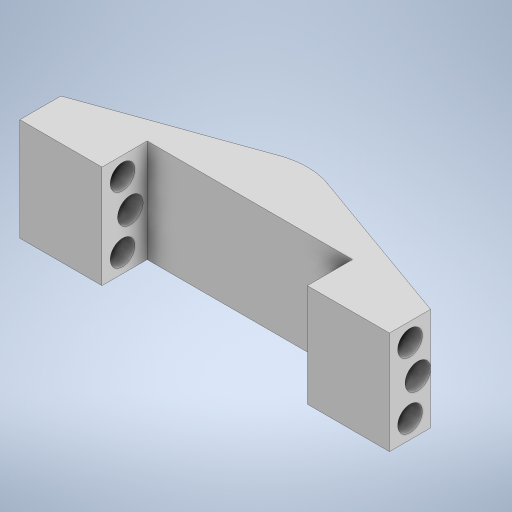
# Autodesk Inventor part: Schieber
Saved by Autodesk Inventor 2024 (Build 280153000, 153)
## iProperties
Created: 2023-08-23
Part Number: Schieber
Material: Generisch
Document SubType Name: Modeling
Designer: rapp
Density: 1 g/cm^3
Appearance: Vorgabe
Author: rapp
Autodesk Inventor part; units mm, degrees
ref_plane "YZ Plane" through (0, 0, 0) normal (1, 0, 0) x (0, 1, 0)
ref_plane "XZ Plane" through (0, 0, 0) normal (0, 1, 0) x (-1, 0, 0)
ref_plane "XY Plane" through (0, 0, 0) normal (0, 0, 1) x (1, 0, 0)
sketch "Skizze1" plane through (0, 0, 0) normal (0, 0, 1) x (1, 0, 0)
  line L0 (-63, 0) -> (63, 0) projected
  line L1 (0, -6) -> (0, 18.5) projected
  arc A0 (5.8901, 13.979) -> (-5.8901, 13.979) centre (0, -2.5) ccw
  line L2 (-5.8901, 13.979) -> (-45, 0)
  line L3 (5.8901, 13.979) -> (45, 0)
  line L4 (-45, 0) -> (45, 0)
  dimension "d2" = 35
  dimension "d3" = 15
  dimension "d4" = 45
  constraints: 6 end point, 2 point on circle, 2 point on line, 2 symmetric about line, 1 centre point, 1 collinear, 1 tangent
  measures "d2" diameter of A0
  measures "d3" distance edge to line of A0 L0
  measures "d4" distance from line of L1 L2.end
extrude "Extrusion1" add sketch "Skizze1" along normal blind 25
sketch "Skizze4" plane through (-45, 0, 0) normal (0, -1, 0) x (1, 0, 0)
  line L0 (0, 25) -> (90, 25) projected
  line L1 (0, 0) -> (0, 25) projected
  line L2 (90, 25) -> (0, 25)
  line L3 (0, 25) -> (0, 0)
  line L4 (0, 0) -> (90, 0)
  line L5 (90, 0) -> (90, 25)
  point P0 (45, 0)
  constraints: 8 end point, 2 parallel, 1 horizontal, 1 perpendicular
extrude "Extrusion4" add sketch "Skizze4" along normal blind 10
sketch "Skizze5" plane through (-45, -10, 0) normal (-1, 0, 0) x (0, 0, 1)
  line L0 (25, 0) -> (0, 0) projected
  line L1 (0, 10) -> (0, 0) projected
  point P0 (4.5, 5)
  point P1 (20.5, 5)
  dimension "d17" = 5
  dimension "d18" = 5
  dimension "d19" = 25
  dimension "d20" = 16
  dimension "d21" = 4.5
  measures "d17" distance from line of point (4.5, 5) L0
  measures "d18" distance from line of point (20.5, 5) L0
  measures "d19" distance of L0.start L0.end
  measures "d20" distance of point (20.5, 5) point (4.5, 5)
  measures "d21" distance from line of L1 point (4.5, 5)
hole "Bohrung1" at (-45, -5, 4.5) at (-45, -5, 20.5) direction (1, 0, 0) diameter 6 end through all
sketch "Skizze6" plane through (-45, -10, 0) normal (-1, 0, 0) x (0, 0, 1)
  line L0 (0, 10) -> (25, 10) projected
  line L1 (0, 23.979) -> (0, 10) projected
  point P0 (12.5, 6.9)
  dimension "d29" = 3.1
  dimension "d30" = 12.5
  measures "d29" distance from line of point (12.5, 6.9) L0
  measures "d30" distance from line of L1 point (12.5, 6.9)
hole "Bohrung2" at (-45, -3.1, 12.5) direction (1, 0, 0) diameter 6.2 end through all
sketch "Skizze7" plane through (0, 0, 0) normal (0, 0, -1) x (-1, 0, 0)
  line L0 (0, -15) -> (0, 20) projected
  line L1 (45, -10) -> (-45, -10) projected
  line L2 (-25, -10) -> (25, -10)
  line L3 (25, -10) -> (25, 1)
  line L4 (25, 1) -> (-25, 1)
  line L5 (-25, 1) -> (-25, -10)
  point P0 (0, 0)
  dimension "d38" = 50
  dimension "d39" = 11
  constraints: 8 end point, 2 parallel, 1 horizontal, 1 perpendicular, 1 point on line, 1 other
  measures "d38" distance of L4.end L3.end
  measures "d39" distance of L3.end L2.end
extrude "Extrusion5" cut sketch "Skizze7" against normal blind 25
